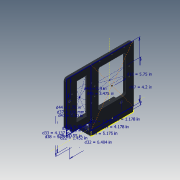
# Autodesk Inventor part: Standard
Saved by Autodesk Inventor 2020.3 (Build 243373000, 373)
## iProperties
RuleStatus: InUse
AfterDocSave0: file://Part Number Cleaner
Created: 2023-02-09
Material: ABS, BLACK
Catalog Web Link: https://www.janelia.org/
Vendor: HHMI: JRC - jET
Document SubType Name: Modeling
Designer: arnoldj
Density: 1.06 g/cm^3
Appearance: Black Anodize
Mass: 108.984 g
Surface Area: 487.943 cm^2
Volume: 108.984 cm^3
DESIGN DEPARTMENT: HHMI: JRC - jET
ALTERED ITEM PART NUMBER: N/A
ALTERED ITEM VENDOR: N/A
ALTERED ITEM DESCRIPTION: N/A
Title: Standard
Author: arnoldj
Revision Number: 0
Autodesk Inventor part; units mm, degrees
ref_plane "YZ Plane" through (0, 0, 0) normal (1, 0, 0) x (0, 1, 0)
ref_plane "XZ Plane" through (0, 0, 0) normal (0, 1, 0) x (-1, 0, 0)
ref_plane "XY Plane" through (0, 0, 0) normal (0, 0, 1) x (1, 0, 0)
sketch "Sketch1" plane through (0, 0, 0) normal (0, 1, 0) x (-1, 0, 0)
  line L0 (0, -75.565) -> (0, 75.565) projected
  line L1 (-9.8806, 0) -> (59.2836, 0) projected
  line L2 (36.703, -40.64) -> (9.525, -40.64)
  line L3 (9.525, -40.64) -> (9.525, 40.64)
  line L4 (9.525, 40.64) -> (36.703, 40.64)
  line L5 (36.703, 40.64) -> (36.703, -40.64)
  line L6 (36.703, -40.64) -> (9.525, 40.64) construction
  line L7 (9.525, -40.64) -> (36.703, 40.64) construction
  line L8 (0, -53.975) -> (49.403, -53.975)
  line L9 (49.403, -53.975) -> (49.403, 53.975)
  line L10 (49.403, 53.975) -> (0, 53.975)
  line L11 (0, 53.975) -> (0, -53.975)
  line L12 (0, -53.975) -> (49.403, 53.975) construction
  line L13 (49.403, -53.975) -> (0, 53.975) construction
  point P0 (0, 0)
  point P1 (23.114, 0)
  point P2 (24.7015, 0)
  dimension "d0" = 81.28
  dimension "d1" = 27.178
  dimension "d3" = 107.95
  dimension "d4" = 12.7
  dimension "d6" = 9.525
  dimension "d7" = 0
  constraints: 24 end point, 5 midpoint, 4 parallel, 2 horizontal, 2 perpendicular, 1 point on line
  measures "d0" distance of L4.end L2.start
  measures "d1" distance of L3.end L4.end
  measures "d3" distance of L8.end L9.end
  measures "d4" distance between parallel lines of L5 L9
  measures "d6" distance between parallel lines of L3 L11
  measures "d7" distance between parallel lines of L11 L0
extrude "Extrusion1" add sketch "Sketch1" against normal blind 12.7 contours L0 L1 L3 L2 L5 L9 L8 | L0 L10 L9 L1 L5 L4 L3
sketch "Sketch2" plane through (0, 0, 0) normal (0, 1, 0) x (1, 0, 0)
  point P0 (0, 0)
sketch "Sketch4" plane through (0, 0, 0) normal (0, 1, 0) x (1, 0, 0)
  point P0 (0, 0)
sketch "Sketch5" plane through (0, 0, 0) normal (0, 1, 0) x (1, 0, 0)
  line L0 (9.8806, 0) -> (-59.2836, 0) projected
  line L1 (0, 75.565) -> (0, -75.565) projected
  line L2 (-39.878, 48.26) -> (-6.223, 48.26)
  line L3 (-6.223, 48.26) -> (-6.223, -48.26)
  line L4 (-6.223, -48.26) -> (-39.878, -48.26)
  line L5 (-39.878, -48.26) -> (-39.878, 48.26)
  line L6 (-39.878, 48.26) -> (-6.223, -48.26) construction
  line L7 (-6.223, 48.26) -> (-39.878, -48.26) construction
  line L8 (-9.525, 40.64) -> (-9.525, -40.64) projected
  point P0 (0, 0)
  point P1 (-23.0505, 0)
  dimension "d13" = 3.302
  dimension "d14" = 96.52
  dimension "d15" = 33.655
  constraints: 12 end point, 2 midpoint, 2 parallel, 1 horizontal, 1 perpendicular, 1 point on line
  measures "d13" distance between parallel lines of L3 L8
  measures "d14" distance of L4.end L2.start
  measures "d15" distance of L3.end L4.end
extrude "Extrusion3" cut sketch "Sketch5" against normal blind 9.525
sketch "Sketch3" plane through (0, 0, 53.975) normal (1, 0, 0) x (0, 0, -1)
  line L0 (0, 0) -> (0, -12.7) projected
  line L1 (0, 0) -> (107.95, 0) projected
  line L2 (107.95, 0) -> (107.95, -12.7) projected
  line L3 (107.95, 146.05) -> (0, 146.05)
  line L4 (0, 146.05) -> (0, 0)
  line L5 (0, 0) -> (107.95, 0)
  line L6 (107.95, 0) -> (107.95, 146.05)
  line L7 (107.95, 146.05) -> (0, 0) construction
  line L8 (0, 146.05) -> (107.95, 0) construction
  line L9 (0, 20.32) -> (-63.5, 20.32)
  line L10 (-63.5, 20.32) -> (-63.5, 146.05)
  line L11 (-63.5, 146.05) -> (0, 146.05)
  line L12 (107.95, -12.7) -> (0, -12.7) projected
  line L13 (-49.53, 20.32) -> (-49.53, 31.75)
  line L14 (-49.53, 31.75) -> (-63.5, 31.75)
  point P0 (53.975, 0)
  point P1 (53.975, 73.025)
  point P2 (1.8288, 24.1808)
  point P3 (78.0288, 24.1808)
  point P4 (-54.7116, 92.3798)
  dimension "d10" = 146.05
  dimension "d18" = 33.02
  dimension "d19" = 63.5
  dimension "d20" = 13.97
  dimension "d21" = 11.43
  dimension "d22" = 36.8808
  dimension "d23" = 29.9212
  dimension "d24" = 106.1212
  dimension "d32" = 162.6616
  dimension "d33" = 105.0798
  constraints: 22 end point, 4 perpendicular, 3 point on line, 2 horizontal, 2 midpoint, 2 parallel, 1 horizontal alignment, 1 vertical
  measures "d10" distance of L3.end L0.start
  measures "d18" distance between parallel lines of L9 L12
  measures "d19" distance of L9.start L9.end
  measures "d20" distance between parallel lines of L10 L13
  measures "d21" distance of L13.start L13.end
  measures "d22" distance from line of point (1.829, 24.181) L12
  measures "d23" distance from line of point (78.029, 24.181) L2
  measures "d24" distance from line of L6 point (1.829, 24.181)
  measures "d32" distance from line of point (-54.712, 92.38) L2
  measures "d33" distance from line of point (-54.712, 92.38) L12
extrude "Extrusion2" add sketch "Sketch3" against normal blind 5.842 contours L4 L3 L6 L1 | L9 L13 L14 L10 L11 L4
hole "Hole1" at (0, 24.1808, -24.0538) at (0, 24.1808, 52.1462) at (0, 92.3798, 108.6866) direction (-1, 0, 0) diameter 6.35 end through all
sketch "Sketch6" plane through (-5.842, 0, 53.975) normal (-1, 0, 0) x (0, 0, 1)
  line L0 (3.495, 135.55) -> (43.495, 135.55)
  line L1 (43.495, 135.55) -> (43.495, 29.55)
  line L2 (43.495, 29.55) -> (3.495, 29.55)
  line L3 (3.495, 29.55) -> (3.495, 135.55)
  line L4 (3.495, 135.55) -> (43.495, 29.55) construction
  line L5 (43.495, 135.55) -> (3.495, 29.55) construction
  line L6 (0, -12.7) -> (-107.95, -12.7) projected
  line L7 (-107.95, 0) -> (-107.95, -12.7) projected
  line L8 (48.575, 104.775) -> (-1.585, 104.775) construction
  line L9 (-1.585, 104.775) -> (-1.585, 60.325) construction
  line L10 (-1.585, 60.325) -> (48.575, 60.325) construction
  line L11 (48.575, 60.325) -> (48.575, 104.775) construction
  line L12 (48.575, 104.775) -> (-1.585, 60.325) construction
  line L13 (-1.585, 104.775) -> (48.575, 60.325) construction
  line L14 (-53.975, 177.8) -> (-53.975, -44.45) construction
  line L15 (-142.24, 0) -> (97.79, 0) construction
  line L16 (-98.1075, 93.98) -> (-9.8425, 93.98) construction
  line L17 (-9.8425, 93.98) -> (-9.8425, 71.12) construction
  line L18 (-9.8425, 71.12) -> (-98.1075, 71.12) construction
  line L19 (-98.1075, 71.12) -> (-98.1075, 93.98) construction
  line L20 (-98.1075, 93.98) -> (-9.8425, 71.12) construction
  line L21 (-9.8425, 93.98) -> (-98.1075, 71.12) construction
  point P0 (-53.975, 0)
  point P1 (23.495, 82.55)
  point P2 (-53.975, 82.55)
  dimension "d36" = 40
  dimension "d37" = 106
  dimension "d38" = 95.25
  dimension "d39" = 131.445
  dimension "d43" = 5.08
  dimension "d44" = 44.45
  dimension "d45" = 88.265
  dimension "d46" = 22.86
  dimension "d47" = 106.68
  constraints: 36 end point, 6 midpoint, 6 parallel, 4 coincident, 3 horizontal, 3 perpendicular, 1 point on line
  measures "d36" distance of L1.end L2.end
  measures "d37" distance of L0.end L1.end
  measures "d38" distance from line of L6 point (23.495, 82.55)
  measures "d39" distance from line of point (23.495, 82.55) L7
  measures "d43" distance between parallel lines of L1 L11
  measures "d44" distance of L10.end L8.start
  measures "d45" distance of L17.end L18.end
  measures "d46" distance of L16.end L17.end
  measures "d47" distance between parallel lines of L6 L16
extrude "Extrusion4" cut sketch "Sketch6" against normal blind 2.54
fillet "Fillet3" radius 1.27 4 edges at (-4.572, 29.55, 97.47) (-4.572, 29.55, 57.47) (-4.572, 135.55, 57.47) (-4.572, 135.55, 97.47)
hole "Hole2" at (-5.842, 93.98, 44.1325) at (-5.842, 71.12, 44.1325) at (-5.842, 71.12, -44.1325) at (-5.842, 93.98, -44.1325) at (-5.842, 104.775, 52.39) at (-5.842, 60.325, 52.39) at (-5.842, 60.325, 102.55) at (-5.842, 104.775, 102.55) direction (1, 0, 0) diameter 2.6416 end through all thread size "6-32 UNC" class "2B" standard "ANSI Unified Screw Threads"
fillet "Fillet1" radius 3.175 2 edges at (-2.921, 31.75, 103.505) (-2.921, 20.32, 103.505)
fillet "Fillet2" radius 12.7 1 edges at (-2.921, 20.32, 53.975)
sketch "Sketch7" plane through (-5.842, 0, 53.975) normal (-1, 0, 0) x (0, 0, 1)
  line L0 (-98.1075, 93.98) -> (-9.8425, 93.98) construction
  circle A0 centre (-9.8425, 93.98) radius 1.3208 construction
  line L1 (-98.1075, 142.24) -> (-9.8425, 142.24) construction
  line L2 (-9.8425, 142.24) -> (-9.8425, 93.98) construction
  line L3 (-9.8425, 93.98) -> (-98.1075, 93.98) construction
  line L4 (-98.1075, 93.98) -> (-98.1075, 142.24) construction
  line L5 (-98.1075, 142.24) -> (-9.8425, 93.98) construction
  line L6 (-9.8425, 142.24) -> (-98.1075, 93.98) construction
  line L7 (63.5, 146.05) -> (-107.95, 146.05) construction
  point P0 (-53.975, 0)
  point P1 (-53.975, 118.11)
  point P2 (-53.975, 142.24)
  point P3 (-22.5425, 142.24)
  point P4 (-85.4075, 142.24)
  dimension "d55" = 3.81
  dimension "d75" = 12.7
  dimension "d76" = 12.7
  constraints: 12 end point, 3 midpoint, 2 coincident, 2 parallel, 2 point on line, 1 horizontal, 1 perpendicular
  measures "d55" distance between parallel lines of L1 L7
  measures "d75" distance of L1.end point (-22.543, 142.24)
  measures "d76" distance of L1.start point (-85.408, 142.24)
hole "Hole3" at (-5.842, 142.24, 0) at (-5.842, 142.24, 31.4325) at (-5.842, 142.24, -31.4325) direction (1, 0, 0) diameter 2.3622 end through all
fillet "Fillet4" radius 6.35 3 edges at (-2.921, 146.05, 117.475) (-2.921, 146.05, -53.975) (-2.921, 31.75, 117.475)
fillet "Fillet5" radius 4.7625 2 edges at (-49.403, -6.35, 53.975) (-49.403, -6.35, -53.975)
sketch "Sketch8" plane through (-5.842, 0, 53.975) normal (-1, 0, 0) x (0, 0, 1)
  line L0 (-88.7872, 129.4659) -> (-18.9372, 129.4659)
  line L1 (-18.9372, 129.4659) -> (-18.9372, 34.8509)
  line L2 (-18.9372, 34.8509) -> (-88.7872, 34.8509)
  line L3 (-88.7872, 34.8509) -> (-88.7872, 129.4659)
  line L4 (-88.7872, 129.4659) -> (-18.9372, 34.8509) construction
  line L5 (-18.9372, 129.4659) -> (-88.7872, 34.8509) construction
  point P0 (-53.975, 0)
  point P1 (-53.8622, 82.1584)
  dimension "d65" = 69.85
  dimension "d66" = 94.615
  constraints: 12 end point, 2 midpoint, 2 parallel, 1 horizontal, 1 perpendicular
  measures "d65" distance of L1.end L2.end
  measures "d66" distance of L2.end L0.start
extrude "Extrusion5" cut sketch "Sketch8" against normal through all
fillet "Fillet6" radius 4.7625 4 edges at (-2.921, 129.4659, 35.0378) (-2.921, 34.8509, -34.8122) (-2.921, 129.4659, -34.8122) (-2.921, 34.8509, 35.0378)
sketch "Sketch9" plane through (-3.302, 0, 53.975) normal (-1, 0, 0) x (0, 0, 1)
  arc A0 (43.495, 134.28) -> (42.225, 135.55) centre (42.225, 134.28) ccw projected
  line L0 (4.765, 135.55) -> (42.225, 135.55) projected
  arc A1 (4.765, 135.55) -> (3.495, 134.28) centre (4.765, 134.28) ccw projected
  line L1 (3.495, 30.82) -> (3.495, 134.28) projected
  arc A2 (3.495, 30.82) -> (4.765, 29.55) centre (4.765, 30.82) ccw projected
  line L2 (42.225, 29.55) -> (4.765, 29.55) projected
  arc A3 (42.225, 29.55) -> (43.495, 30.82) centre (42.225, 30.82) ccw projected
  line L3 (43.495, 134.28) -> (43.495, 30.82) projected
  line L4 (11.0923, 37.1473) -> (11.0923, 127.9527)
  line L5 (11.0923, 127.9527) -> (35.8977, 127.9527)
  line L6 (35.8977, 127.9527) -> (35.8977, 37.1473)
  line L7 (35.8977, 37.1473) -> (11.0923, 37.1473)
  point P0 (-53.975, 0)
  point P1 (23.495, 82.55)
  constraints: 8 end point, 3 other
extrude "Extrusion6" cut sketch "Sketch9" against normal through all contours L4 L5 L6 L7
chamfer "Chamfer1" distance 3.175 angle 45 5 edges at (-25.2413, 0, -53.975) (-48.0081, 0, -52.5801) (-49.403, 0, 0) (-48.0081, 0, 52.5801) (-25.2412, 0, 53.975)
fillet "Fillet7" radius 4.7625 4 edges at (-36.703, -11.1125, 40.64) (-9.525, -11.1125, 40.64) (-9.525, -11.1125, -40.64) (-36.703, -11.1125, -40.64)
body "Solid1"
